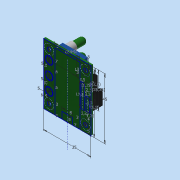
# Autodesk Inventor part: Motherboard_dummy
Saved by Autodesk Inventor 2015 (Build 190159000, 159)
## iProperties
Created: 2014-12-25
Part Number: Motherboard_dummy
Material: ABS Plastic
Document SubType Name: Modeling
Designer: Openlab
Density: 1.06 g/cm^3
Appearance: Smooth - Dark Forest Green
Mass: 9.08054 g
Surface Area: 59.127 cm^2
Volume: 8.56654 cm^3
Author: Openlab
Autodesk Inventor part; units mm, degrees
ref_plane "YZ Plane" through (0, 0, 0) normal (1, 0, 0) x (0, 1, 0)
ref_plane "XZ Plane" through (0, 0, 0) normal (0, 1, 0) x (-1, 0, 0)
ref_plane "XY Plane" through (0, 0, 0) normal (0, 0, 1) x (1, 0, 0)
sketch "Sketch1" plane through (0, 0, 0) normal (0, 1, 0) x (-1, 0, 0)
  line L0 (0, 0) -> (0, 45)
  line L1 (35, 45) -> (35, 0)
  line L2 (35, 0) -> (0, 0)
  line L3 (0, 45) -> (35, 45)
  line L4 (26.771, 0) -> (8.229, 0)
  line L5 (8.229, 0) -> (8.229, 43.18)
  line L6 (8.229, 43.18) -> (26.771, 43.18)
  line L7 (26.771, 43.18) -> (26.771, 0)
  line L8 (17.5, -18.3373) -> (17.5, 40.4461) construction
  line L9 (13.5, 5) -> (21.5, 5)
  line L10 (21.5, 5) -> (21.5, 0)
  line L11 (21.5, 0) -> (13.5, 0)
  line L12 (13.5, 0) -> (13.5, 5)
  circle A0 centre (31, 40) radius 1.5
  circle A1 centre (4, 40) radius 1.5
  circle A2 centre (31, 5) radius 1.5
  circle A3 centre (4, 5) radius 1.5
  line L13 (5, 13.75) -> (5, 31.25)
  line L14 (5, 31.25) -> (7.5, 31.25)
  line L15 (7.5, 31.25) -> (7.5, 13.75)
  line L16 (7.5, 13.75) -> (5, 13.75)
  line L17 (1.25, 13.75) -> (1.25, 23.75)
  line L18 (1.25, 23.75) -> (3.75, 23.75)
  line L19 (3.75, 23.75) -> (3.75, 13.75)
  line L20 (3.75, 13.75) -> (1.25, 13.75)
  circle A4 centre (31, 33) radius 3
  circle A5 centre (31, 33) radius 2.5
  circle A6 centre (31, 23) radius 3
  circle A7 centre (31, 23) radius 2.5
  circle A8 centre (31, 13) radius 3
  circle A9 centre (31, 13) radius 2.5
  circle A10 centre (4, 5) radius 3.5 construction
  circle A11 centre (4, 40) radius 3.5 construction
  line L21 (4.7146, 22.5) -> (8.1867, 22.5) construction
  line L22 (0.8216, 18.75) -> (4.7146, 18.75) construction
  circle A12 centre (31, 40) radius 3.5 construction
  circle A13 centre (31, 5) radius 3.5 construction
  line L23 (6.25, 31.7194) -> (6.25, 13) construction
  line L24 (2.5, 24.6777) -> (2.5, 12.6859) construction
  point P0 (17.5, 0)
  point P1 (17.5, 0)
  dimension "d42" = 5
  dimension "d43" = 5
  dimension "d44" = 4
  dimension "d45" = 4
  dimension "d47" = 18.542
  dimension "d49" = 43.18
  dimension "d50" = 5
  dimension "d51" = 8
  dimension "d52" = 35
  dimension "d53" = 45
  dimension "d54" = 3
  dimension "d55" = 3
  dimension "d56" = 3
  dimension "d57" = 3
  dimension "d59" = 2.5
  dimension "d66" = 10
  dimension "d67" = 10
  dimension "d68" = 6
  dimension "d69" = 5
  dimension "d70" = 6
  dimension "d71" = 5
  dimension "d72" = 6
  dimension "d73" = 5
  dimension "d76" = 12
  dimension "d81" = 7
  dimension "d82" = 7
  dimension "d85" = 17.5
  dimension "d87" = 7
  dimension "d88" = 7
  dimension "d89" = 2.5
  dimension "d90" = 10
  dimension "d91" = 1.25
  dimension "d92" = 1.25
  dimension "d93" = 22.5
  dimension "d94" = 26.25
  dimension "d95" = 6.25
  dimension "d96" = 2.5
  constraints: 50 end point, 19 coincident, 14 centre point, 11 perpendicular, 5 vertical alignment, 3 collinear, 3 horizontal alignment, 2 horizontal, 2 vertical, 1 midpoint, 8 other
  measures "d42" distance from line of L3 A1.centre
  measures "d43" distance from line of L2 A3.centre
  measures "d44" distance from line of L0 A3.centre
  measures "d45" distance from line of L1 A2.centre
  measures "d47" distance of L6.start L6.end
  measures "d49" distance of L4.end L6.start
  measures "d50" distance of L11.end L9.start
  measures "d51" distance of L9.start L9.end
  measures "d52" distance of L2.start L2.end
  measures "d53" distance of L2.end L3.start
  measures "d54" diameter of A3
  measures "d55" diameter of A1
  measures "d56" diameter of A2
  measures "d57" diameter of A0
  measures "d59" distance of L14.start L14.end
  measures "d66" distance of point (31, 23) point (31, 13)
  measures "d67" distance of point (31, 33) point (31, 23)
  measures "d68" diameter of A4
  measures "d69" diameter of A5
  measures "d70" diameter of A6
  measures "d71" diameter of A7
  measures "d72" diameter of A8
  measures "d73" diameter of A9
  measures "d76" distance from line of L3 A4.centre
  measures "d81" diameter of A10
  measures "d82" diameter of A11
  measures "d85" distance of L14.end L15.end
  measures "d87" diameter of A12
  measures "d88" diameter of A13
  measures "d89" distance of L18.start L18.end
  measures "d90" distance of L17.start L18.start
  measures "d91" distance between parallel lines of L0 L17
  measures "d92" distance between parallel lines of L19 L13
  measures "d93" distance between parallel lines of L3 L21
  measures "d94" distance between parallel lines of L3 L22
  measures "d95" distance between parallel lines of L0 L23
  measures "d96" distance between parallel lines of L0 L24
extrude "Extrusion1" add sketch "Sketch1" along normal blind 1.5 contours L0 L3 L1 L2 L7 L6 L5 | L5 L6 L7 L2 L10 L9 L12 | L12 L9 L10 L2 | L13 L14 L15 L16 | L17 L18 L19 L20 | A4 | A5 | A6 | A7 | A8 | A9
extrude "Extrusion2" add sketch "Sketch1" along normal blind 6 contours L5 L6 L7 L2 L10 L9 L12 | L12 L9 L10 L2
extrude "Extrusion3" add sketch "Sketch1" along normal blind 10 contours L12 L9 L10 L2
extrude "Extrusion4" add sketch "Sketch1" along normal blind 10 contours L13 L14 L15 L16 | L17 L18 L19 L20
extrude "Extrusion5" add sketch "Sketch1" along normal blind 26.5 contours A5 | A7 | A9
fillet "Fillet1" radius 2.5 3 edges at (-28.5, 26.5, 33) (-28.5, 26.5, 23) (-28.5, 26.5, 13)
extrude "Extrusion6" add sketch "Sketch1" along normal blind 18 contours A4 | A6 | A8
sketch "Sketch2" plane through (0, 0, 0) normal (0, 0, -1) x (-1, 0, 0)
  line L0 (13.5, 10) -> (21.5, 10)
  line L1 (21.5, 10) -> (21.5, 6)
  line L2 (21.5, 6) -> (13.5, 6)
  line L3 (13.5, 6) -> (13.5, 10)
  line L4 (17.5, 0) -> (17.5, 11.1987) construction
  line L5 (0, 0) -> (35, 0) projected
  dimension "d99" = 6
  dimension "d100" = 4
  dimension "d101" = 8
  constraints: 10 end point, 2 parallel, 2 perpendicular, 1 horizontal, 1 midpoint, 1 vertical, 1 other
  measures "d99" distance from line of L5.start L2
  measures "d100" distance of L2.end L0.start
  measures "d101" distance of L0.start L0.end
extrude "Extrusion7" add sketch "Sketch2" along normal blind 1.5
body "Solid1"
